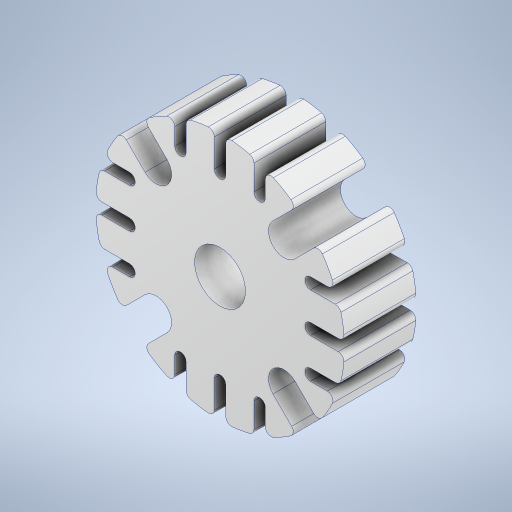
# Autodesk Inventor part: Hotend Spacer
Saved by Autodesk Inventor 2024 (Build 280153000, 153)
## iProperties
Created: 2025-01-03
Part Number: Hotend Spacer
Material: Aluminum 6061
Document SubType Name: Modeling
Designer: Ishaan
Density: 2.7 g/cm^3
Appearance: Aluminum - Flat
Author: Ishaan
Autodesk Inventor part; units mm, degrees
ref_plane "YZ Plane" through (0, 0, 0) normal (1, 0, 0) x (0, 1, 0)
ref_plane "XZ Plane" through (0, 0, 0) normal (0, 1, 0) x (-1, 0, 0)
ref_plane "XY Plane" through (0, 0, 0) normal (0, 0, 1) x (1, 0, 0)
sketch "Sketch1" plane through (0, 0, 0) normal (0, 0, 1) x (1, 0, 0)
  circle A0 centre (0, 0) radius 11
  circle A1 centre (0, 0) radius 8 construction
  line L0 (5.6569, -5.6569) -> (-5.6569, -5.6569) construction
  line L1 (-5.6569, -5.6569) -> (-5.6569, 5.6569) construction
  line L2 (-5.6569, 5.6569) -> (5.6569, 5.6569) construction
  line L3 (5.6569, 5.6569) -> (5.6569, -5.6569) construction
  line L4 (5.6569, -5.6569) -> (-5.6569, 5.6569) construction
  line L5 (-5.6569, -5.6569) -> (5.6569, 5.6569) construction
  line L6 (-5.6569, 5.6569) -> (-7.7782, 7.7782) construction
  line L7 (-4.6846, 6.6291) -> (-6.8059, 8.7504)
  line L8 (-8.7504, 6.8059) -> (-6.6291, 4.6846)
  arc A2 (-6.6291, 4.6846) -> (-4.6846, 6.6291) centre (-5.6569, 5.6569) ccw
  arc A3 (-6.8059, 8.7504) -> (-8.7504, 6.8059) centre (-7.7782, 7.7782) ccw
  line L9 (-5.6569, -5.6569) -> (-7.7782, -7.7782) construction
  line L10 (-6.6291, -4.6846) -> (-8.7504, -6.8059)
  line L11 (-6.8059, -8.7504) -> (-4.6846, -6.6291)
  arc A4 (-4.6846, -6.6291) -> (-6.6291, -4.6846) centre (-5.6569, -5.6569) ccw
  arc A5 (-8.7504, -6.8059) -> (-6.8059, -8.7504) centre (-7.7782, -7.7782) ccw
  line L12 (5.6569, -5.6569) -> (7.7782, -7.7782) construction
  line L13 (4.6846, -6.6291) -> (6.8059, -8.7504)
  line L14 (8.7504, -6.8059) -> (6.6291, -4.6846)
  arc A6 (6.6291, -4.6846) -> (4.6846, -6.6291) centre (5.6569, -5.6569) ccw
  arc A7 (6.8059, -8.7504) -> (8.7504, -6.8059) centre (7.7782, -7.7782) ccw
  line L15 (5.6569, 5.6569) -> (7.7782, 7.7782) construction
  line L16 (6.6291, 4.6846) -> (8.7504, 6.8059)
  line L17 (6.8059, 8.7504) -> (4.6846, 6.6291)
  arc A8 (4.6846, 6.6291) -> (6.6291, 4.6846) centre (5.6569, 5.6569) ccw
  arc A9 (8.7504, 6.8059) -> (6.8059, 8.7504) centre (7.7782, 7.7782) ccw
  circle A10 centre (0, 0) radius 2.25
  point P0 (-6.7175, 6.7175)
  point P1 (-6.7175, -6.7175)
  point P2 (6.7175, -6.7175)
  point P3 (6.7175, 6.7175)
  point P4 (-8.6894, 6.7449)
  point P5 (-8.6894, -6.7449)
  point P6 (-6.7449, -8.6894)
  point P7 (6.7449, -8.6894)
  point P8 (8.6894, -6.7449)
  point P9 (8.6894, 6.7449)
  point P10 (6.7449, 8.6894)
  point P11 (-6.7449, 8.6894)
  dimension "d0" = 22
  dimension "d1" = 16
  dimension "d2" = 2.75
  dimension "d5" = 360
  dimension "d7" = 4.5
  constraints: 44 end point, 16 point on circle, 9 centre point, 4 tangent, 3 coincident, 3 midpoint, 3 parallel, 2 perpendicular, 1 collinear, 1 horizontal, 55 other
  measures "d2" diameter of A3
  measures "d7" diameter of A10
extrude "Extrusion1" add sketch "Sketch1" along normal blind 6.35 contours A0 L14 A6 L13 L11 A4 L10 L8 A2 L7 L17 A8 L16
fillet "Fillet1" radius 0.5 8 edges at (-8.6894, 6.7449, 3.175) (-8.6894, -6.7449, 3.175) (-6.7449, -8.6894, 3.175) (6.7449, -8.6894, 3.175) (8.6894, 6.7449, 3.175) (-6.7449, 8.6894, 3.175) (8.6894, -6.7449, 3.175) (6.7449, 8.6894, 3.175)
sketch "Sketch2" plane through (0, 0, 6.35) normal (0, 0, 1) x (1, 0, 0)
  line L0 (-11, 3.5) -> (-8, 3.5) construction
  line L1 (-11, 3) -> (-8, 3)
  line L2 (-8, 4) -> (-11, 4)
  arc A0 (-11, 4) -> (-11, 3) centre (-11, 3.5) ccw
  arc A1 (-8, 3) -> (-8, 4) centre (-8, 3.5) ccw
  line L3 (-8, 0) -> (-11, 0) construction
  line L4 (-8, 0.5) -> (-11, 0.5)
  line L5 (-11, -0.5) -> (-8, -0.5)
  arc A2 (-8, -0.5) -> (-8, 0.5) centre (-8, 0) ccw
  arc A3 (-11, 0.5) -> (-11, -0.5) centre (-11, 0) ccw
  line L6 (-8, -3.5) -> (-11, -3.5) construction
  line L7 (-8, -4) -> (-11, -4)
  line L8 (-11, -3) -> (-8, -3)
  arc A4 (-8, -4) -> (-8, -3) centre (-8, -3.5) ccw
  arc A5 (-11, -3) -> (-11, -4) centre (-11, -3.5) ccw
  arc A6 (-9.0421, 6.2642) -> (-9.0421, -6.2642) centre (0, 0) ccw projected
  point P0 (-9.5, 3.5)
  point P1 (-9.5, 0)
  point P2 (-9.5, -3.5)
  point P3 (-10.247, 4)
  point P4 (-10.583, 3)
  point P5 (-10.9886, 0.5)
  point P6 (-10.9886, -0.5)
  point P7 (-10.583, -3)
  point P8 (-10.247, -4)
  dimension "d11" = 1
  dimension "d12" = 3
  dimension "d13" = 2.5
  dimension "d14" = 2.5
  constraints: 24 end point, 13 point on circle, 12 tangent, 6 centre point, 6 parallel, 3 midpoint, 2 equal radius, 2 horizontal, 2 vertical alignment, 1 point on line
  measures "d11" diameter of A1
  measures "d12" distance of L3.start L3.end
  measures "d13" distance between parallel lines of L4 L1
  measures "d14" distance between parallel lines of L8 L5
extrude "Extrusion2" cut sketch "Sketch2" against normal through all contours A6 L2 A1 L1 | A2 L5 A6 L4 | L7 A6 L8 A4
pattern_circular "Circular Pattern1" count 4 over 360 about axis through (0, 0, 0) along (0, 0, 1) of "Extrusion2"
fillet "Fillet2" radius 0.5 24 edges at (10.9886, -0.5, 3.175) (10.9886, 0.5, 3.175) (10.583, -3, 3.175) (10.247, -4, 3.175) (4, -10.247, 3.175) (3, -10.583, 3.175) (10.583, 3, 3.175) (10.247, 4, 3.175) (0.5, 10.9886, 3.175) (3, 10.583, 3.175) (4, 10.247, 3.175) (0.5, -10.9886, 3.175) (-0.5, -10.9886, 3.175) (-3, -10.583, 3.175) (-4, -10.247, 3.175) (-10.247, -4, 3.175) (-10.583, -3, 3.175) (-10.9886, -0.5, 3.175) (-10.9886, 0.5, 3.175) (-10.583, 3, 3.175) (-10.247, 4, 3.175) (-0.5, 10.9886, 3.175) (-3, 10.583, 3.175) (-4, 10.247, 3.175)
equation "\"d14\" = d13"
body "Solid1"
